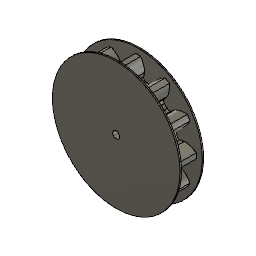
Pinion (12 teeth) (Autodesk Fusion 360 archive; units mm, degrees)
design "Pinion (12 teeth)"
description: Spur Gear; Module: 6.0; Num Teeth: 12; Pressure Angle: 20.0; Backlash: 0.00 mm
part number: Configuration 2
Autodesk Fusion 360 part; units mm, degrees
sketch "Base Circle" plane through (0, 0, 0) normal (0, 0, 1) x (1, 0, 0)
  circle A0 centre (0, 0) radius 29.058
  circle A1 centre (0, 0) radius 2.5
  dimension "dBore" = 5
  measures "dBore" diameter of A1
extrude "Extrude1" add sketch "Base Circle" along normal blind 17
sketch "Gear Tooth" plane through (0, 0, 0) normal (0, 0, 1) x (1, 0, 0)
  spline S0 degree 5 poles (33.47, -4.9149) (33.4943, -4.9185) (33.543, -4.9249) (33.6161, -4.932) (33.714, -4.9371) (33.8368, -4.9373) (33.96, -4.9332) (34.0834, -4.9264) (34.2068, -4.9182) (34.3304, -4.9091) (34.454, -4.8988) (34.5776, -4.8871) (34.7013, -4.8735) (34.8251, -4.8577) (34.949, -4.8398) (35.0728, -4.8198) (35.1967, -4.7983) (35.3206, -4.7752) (35.4445, -4.751) (35.5683, -4.7256) (35.6921, -4.699) (35.8159, -4.6711) (35.9396, -4.6419) (36.0632, -4.6113) (36.1868, -4.5793) (36.3104, -4.5461) (36.4339, -4.5117) (36.5573, -4.4761) (36.6806, -4.4394) (36.8038, -4.4016) (36.927, -4.3627) (37.05, -4.3226) (37.173, -4.2815) (37.2958, -4.2393) (37.4185, -4.1961) (37.5411, -4.1517) (37.6636, -4.1064) (37.7859, -4.06) (37.9082, -4.0126) (38.0302, -3.9642) (38.1522, -3.9148) (38.274, -3.8645) (38.3956, -3.8132) (38.5172, -3.7609) (38.6385, -3.7077) (38.7597, -3.6535) (38.8807, -3.5984) (39.0016, -3.5424) (39.1223, -3.4854) (39.2428, -3.4276) (39.3631, -3.3689) (39.4833, -3.3092) (39.6032, -3.2487) (39.723, -3.1873) (39.8426, -3.125) (39.962, -3.0619) (40.0812, -2.9979) (40.2002, -2.9331) (40.319, -2.8674) (40.4376, -2.8009) (40.5559, -2.7335) (40.6741, -2.6653) (40.792, -2.5963) (40.9098, -2.5265) (41.0273, -2.4559) (41.1445, -2.3844) (41.2616, -2.3122) (41.3783, -2.2392) (41.4949, -2.1654) (41.6112, -2.0908) (41.7273, -2.0154) (41.82, -1.9545) (41.8894, -1.9084) (41.9356, -1.8776) (41.9587, -1.8621) knots 0 0 0 0 0 0 0.01428571 0.02857143 0.04285714 0.05714286 0.07142857 0.08571429 0.1 0.11428571 0.12857143 0.14285714 0.15714286 0.17142857 0.18571429 0.2 0.21428571 0.22857143 0.24285714 0.25714286 0.27142857 0.28571429 0.3 0.31428571 0.32857143 0.34285714 0.35714286 0.37142857 0.38571429 0.4 0.41428571 0.42857143 0.44285714 0.45714286 0.47142857 0.48571429 0.5 0.51428571 0.52857143 0.54285714 0.55714286 0.57142857 0.58571429 0.6 0.61428571 0.62857143 0.64285714 0.65714286 0.67142857 0.68571429 0.7 0.71428571 0.72857143 0.74285714 0.75714286 0.77142857 0.78571429 0.8 0.81428571 0.82857143 0.84285714 0.85714286 0.87142857 0.88571429 0.9 0.91428571 0.92857143 0.94285714 0.95714286 0.97142857 0.98571429 1 1 1 1 1 1
  spline S1 degree 5 poles (33.47, 4.9149) (33.4943, 4.9185) (33.543, 4.9249) (33.6161, 4.932) (33.714, 4.9371) (33.8368, 4.9373) (33.96, 4.9332) (34.0834, 4.9264) (34.2068, 4.9182) (34.3304, 4.9091) (34.454, 4.8988) (34.5776, 4.8871) (34.7013, 4.8735) (34.8251, 4.8577) (34.949, 4.8398) (35.0728, 4.8198) (35.1967, 4.7983) (35.3206, 4.7752) (35.4445, 4.751) (35.5683, 4.7256) (35.6921, 4.699) (35.8159, 4.6711) (35.9396, 4.6419) (36.0632, 4.6113) (36.1868, 4.5793) (36.3104, 4.5461) (36.4339, 4.5117) (36.5573, 4.4761) (36.6806, 4.4394) (36.8038, 4.4016) (36.927, 4.3627) (37.05, 4.3226) (37.173, 4.2815) (37.2958, 4.2393) (37.4185, 4.1961) (37.5411, 4.1517) (37.6636, 4.1064) (37.7859, 4.06) (37.9082, 4.0126) (38.0302, 3.9642) (38.1522, 3.9148) (38.274, 3.8645) (38.3956, 3.8132) (38.5172, 3.7609) (38.6385, 3.7077) (38.7597, 3.6535) (38.8807, 3.5984) (39.0016, 3.5424) (39.1223, 3.4854) (39.2428, 3.4276) (39.3631, 3.3689) (39.4833, 3.3092) (39.6032, 3.2487) (39.723, 3.1873) (39.8426, 3.125) (39.962, 3.0619) (40.0812, 2.9979) (40.2002, 2.9331) (40.319, 2.8674) (40.4376, 2.8009) (40.5559, 2.7335) (40.6741, 2.6653) (40.792, 2.5963) (40.9098, 2.5265) (41.0273, 2.4559) (41.1445, 2.3844) (41.2616, 2.3122) (41.3783, 2.2392) (41.4949, 2.1654) (41.6112, 2.0908) (41.7273, 2.0154) (41.82, 1.9545) (41.8894, 1.9084) (41.9356, 1.8776) (41.9587, 1.8621) knots 0 0 0 0 0 0 0.01428571 0.02857143 0.04285714 0.05714286 0.07142857 0.08571429 0.1 0.11428571 0.12857143 0.14285714 0.15714286 0.17142857 0.18571429 0.2 0.21428571 0.22857143 0.24285714 0.25714286 0.27142857 0.28571429 0.3 0.31428571 0.32857143 0.34285714 0.35714286 0.37142857 0.38571429 0.4 0.41428571 0.42857143 0.44285714 0.45714286 0.47142857 0.48571429 0.5 0.51428571 0.52857143 0.54285714 0.55714286 0.57142857 0.58571429 0.6 0.61428571 0.62857143 0.64285714 0.65714286 0.67142857 0.68571429 0.7 0.71428571 0.72857143 0.74285714 0.75714286 0.77142857 0.78571429 0.8 0.81428571 0.82857143 0.84285714 0.85714286 0.87142857 0.88571429 0.9 0.91428571 0.92857143 0.94285714 0.95714286 0.97142857 0.98571429 1 1 1 1 1 1
  arc A0 (41.9587, -1.8621) -> (41.9587, 1.8621) centre (0, 0) ccw
  line L0 (28.7398, -4.2203) -> (33.47, -4.9149)
  line L1 (28.7398, 4.2203) -> (33.47, 4.9149)
  line L2 (28.7398, -4.2203) -> (28.7398, 4.2203)
  point P0 (34.058, -4.9275)
  point P1 (34.6545, -4.8784)
  point P2 (35.2564, -4.787)
  point P3 (35.862, -4.66)
  point P4 (36.4705, -4.5009)
  point P5 (37.0809, -4.3121)
  point P6 (37.6927, -4.0952)
  point P7 (38.305, -3.8513)
  point P8 (38.9173, -3.5813)
  point P9 (39.5291, -3.286)
  point P10 (40.1396, -2.966)
  point P11 (40.7485, -2.6217)
  point P12 (41.355, -2.2536)
  point P13 (34.058, 4.9275)
  point P14 (34.6545, 4.8784)
  point P15 (35.2564, 4.787)
  point P16 (35.862, 4.66)
  point P17 (36.4705, 4.5009)
  point P18 (37.0809, 4.3121)
  point P19 (37.6927, 4.0952)
  point P20 (38.305, 3.8513)
  point P21 (38.9173, 3.5813)
  point P22 (39.5291, 3.286)
  point P23 (40.1396, 2.966)
  point P24 (40.7485, 2.6217)
  point P25 (41.355, 2.2536)
extrude "Extrude2" add sketch "Gear Tooth" along normal up to surface (17 mm away)
fillet "Fillet1" radius 2 2 edges at (28.7497, -4.2218, 8.5) (28.7497, 4.2218, 8.5)
pattern_circular "C-Pattern1" count 12 over 360 about axis through (0, 0, 0) along (0, 0, 1) of "Extrude2", "Fillet1"
sketch "Diametrial Pitch Circle" plane through (0, 0, 0) normal (0, 0, 1) x (1, 0, 0)
  circle A0 centre (0, 0) radius 36 construction
sketch "Sketch4" plane through (0, 0, 0) normal (1, 0, 0) x (0, 0, -1)
  line L0 (0, 0) -> (0, 46) construction
  line L1 (0, 0) -> (-3, 0)
  line L2 (-3, 0) -> (-0.9916, 46) construction
  line L3 (0, 46) -> (-0.9916, 46)
  line L4 (0, 0) -> (-17, 0) construction
  line L5 (-17, 0) -> (-17, 46) construction
  line L6 (-17, 0) -> (-14, 0) construction
  line L7 (-14, 0) -> (-16.0084, 46) construction
  line L8 (-17, 46) -> (-16.0084, 46)
  line L9 (0, 0) -> (0, 2.5) construction
  line L10 (-17, 0) -> (-17, 2.5) construction
  line L11 (0, 2.5) -> (-2.8908, 2.5)
  line L12 (-0.9916, 46) -> (-2.8908, 2.5)
  line L13 (0, 2.5) -> (0, 46)
  line L14 (-17, 2.5) -> (-14.1092, 2.5)
  line L15 (-14.1092, 2.5) -> (-16.0084, 46)
  line L16 (-17, 46) -> (-17, 2.5)
  dimension "d17" = 3
  dimension "d18" = 46
  dimension "d20" = 17
  dimension "flangeTaper" = 92.5
  dimension "d22" = 3
  dimension "d24" = 92.5
  dimension "d25" = 2.5
  dimension "d26" = 2.5
  constraint coincident L0.start L1.start
  constraint vertical L0
  constraint perpendicular L0 L1
  constraint perpendicular L0 L3
  constraint perpendicular L0 L4
  constraint perpendicular L4 L5
  constraint perpendicular L5 L6
  constraint perpendicular L5 L8
  constraint equal L0 L5
  constraint perpendicular L1 L9
  constraint perpendicular L6 L10
  constraint coincident L2 L11.end
  constraint perpendicular L9 L11
  constraint coincident L7 L14.end
  constraint perpendicular L10 L14
  measures "d17" distance of L0.start L1.end
  measures "d18" distance of L0.start L0.end
  measures "d20" distance of L0.start L4.end
  measures "flangeTaper" angle of L2 L4
  measures "d22" distance of L4.end L6.end
  measures "d24" angle of L4 L7
  measures "d25" distance of L0.start L9.end
  measures "d26" distance of L4.end L10.end
revolve "Revolve1" add sketch "Sketch4" angle 360 about axis through (0, 0, 1.75) along (0, 0, 1)
equation "dThickness = 17 mm"
equation "d18 = ( 92 / 2 ) * 1 mm"
equation "d20 = dThickness"
equation "d24 = flangeTaper"
equation "d25 = dBore / 2"
equation "d26 = dBore / 2"
named bodies: "Spur Gear (12 teeth)"
